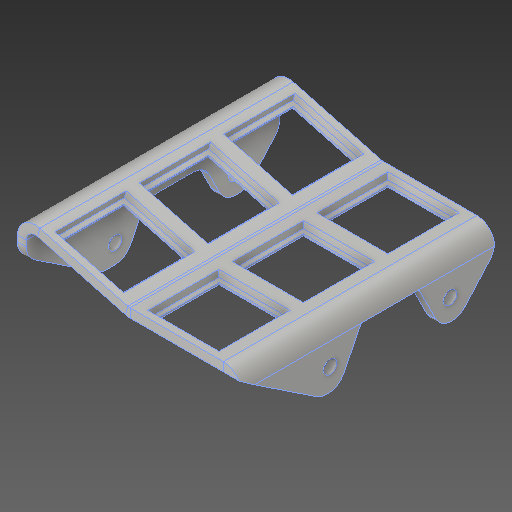
# Autodesk Inventor part: keyplate2
Saved by Autodesk Inventor 2018 (Build 220112000, 112)
## iProperties
Created: 2018-05-25
Part Number: keyplate2
Material: アルミニウム 6061
Document SubType Name: Sheet Metal
Designer: NaMACHAN
Mass: 12.3776 g
Surface Area: 65.0892 cm^2
Volume: 4.58428 cm^3
Density: 2.7 g/cm^3
Flat Pattern Width: 5.7 cm
Flat Pattern Length: 7.68162 cm
Flat Pattern Area: 43.7853 cm^2
Sheet Metal Rule: Al2mm
Sheet Metal Width: 57.000 mm
Sheet Metal Length: 76.816 mm
Sheet Metal Area: 4378.526 mm^2
Appearance: アルミニウム - フラット
Author: NaMACHAN
Autodesk Inventor part; units mm, degrees
ref_plane "YZ Plane" through (0, 0, 0) normal (1, 0, 0) x (0, 1, 0)
ref_plane "XZ Plane" through (0, 0, 0) normal (0, 1, 0) x (-1, 0, 0)
ref_plane "XY Plane" through (0, 0, 0) normal (0, 0, 1) x (1, 0, 0)
sketch "スケッチ1" plane through (0, 0, 0) normal (0, 1, 0) x (-1, 0, 0)
  line L0 (-10.5, -28.5) -> (10.5, -28.5)
  line L1 (10.5, -28.5) -> (10.5, 28.5)
  line L2 (10.5, 28.5) -> (-10.5, 28.5)
  line L3 (-10.5, 28.5) -> (-10.5, -28.5)
  line L4 (-10.5, -28.5) -> (10.5, 28.5) construction
  line L5 (10.5, -28.5) -> (-10.5, 28.5) construction
  line L6 (-7, -7) -> (7, -7)
  line L7 (7, -7) -> (7, 7)
  line L8 (7, 7) -> (-7, 7)
  line L9 (-7, 7) -> (-7, -7)
  line L10 (-7, -7) -> (7, 7) construction
  line L11 (7, -7) -> (-7, 7) construction
  line L12 (-7, -26) -> (7, -26)
  line L13 (7, -26) -> (7, -12)
  line L14 (7, -12) -> (-7, -12)
  line L15 (-7, -12) -> (-7, -26)
  line L16 (-7, -26) -> (7, -12) construction
  line L17 (7, -26) -> (-7, -12) construction
  line L18 (-7, 12) -> (7, 12)
  line L19 (7, 12) -> (7, 26)
  line L20 (7, 26) -> (-7, 26)
  line L21 (-7, 26) -> (-7, 12)
  line L22 (-7, 12) -> (7, 26) construction
  line L23 (7, 12) -> (-7, 26) construction
  point P0 (0, 0)
  point P1 (0, 0)
  point P2 (0, 0)
  point P3 (0, -19)
  point P4 (0, -19)
  point P5 (0, 19)
  point P6 (0, 19)
  point P7 (0, 0)
  dimension "d0" = 21
  dimension "d1" = 57
  dimension "d2" = 14
  dimension "d3" = 14
  dimension "d345" = 14
  dimension "d346" = 14
  dimension "d347" = 14
  dimension "d348" = 14
  dimension "d350" = 19
  dimension "d351" = 19
  measures "d0" distance of L2.end L1.end
  measures "d1" distance of L1.end L0.end
  measures "d2" distance of L8.end L7.end
  measures "d3" distance of L7.end L6.end
  measures "d345" distance of L14.end L13.end
  measures "d346" distance of L13.end L12.end
  measures "d347" distance of L20.end L19.end
  measures "d348" distance of L19.end L18.end
  measures "d350" distance of point (0, -19) point (0, 0)
  measures "d351" distance of point (0, 0) point (0, 19)
extrude "プレート1" add sketch "スケッチ1" along normal blind 2
sketch "スケッチ2" plane through (-11.0176, 2.0681, 28.5) normal (-0.258819, -0.9659258, 0) x (0.9659258, -0.258819, 0)
  line L0 (0, -57) -> (0, 0)
  line L1 (0, 0) -> (-20.4734, 0)
  line L2 (-20.4734, 0) -> (-20.4734, -57)
  line L3 (-20.4734, -57) -> (0, -57)
  constraints: 6 end point, 1 horizontal, 1 perpendicular, 1 vertical
edge flange "フランジ1" height 21 angle 15 thickness 2 bend radius 2 thickness toward (-0.258819, -0.9659258, 0) relief straight relief width 2 relief depth 1 edges at (-10.5, 2, 0) wall of the first edge with corners at (-11.0176, 2.0681, -28.5) (-11.0176, 2.0681, 28.5) (-30.7934, 7.3671, 28.5) (-30.7934, 7.3671, -28.5)
bend "曲げ1"
corner "コーナー1"
sketch "スケッチ9" plane through (-11.0176, 2.0681, 28.5) normal (0.258819, 0.9659258, 0) x (0.9659258, -0.258819, 0)
  line L0 (-17.5, 35.5) -> (-3.5, 35.5)
  line L1 (-3.5, 35.5) -> (-3.5, 21.5)
  line L2 (-3.5, 21.5) -> (-17.5, 21.5)
  line L3 (-17.5, 21.5) -> (-17.5, 35.5)
  line L4 (-17.5, 35.5) -> (-3.5, 21.5) construction
  line L5 (-3.5, 35.5) -> (-17.5, 21.5) construction
  line L6 (-20.4734, 0) -> (0, 0) projected
  line L7 (-20.4734, 57) -> (-20.4734, 0) projected
  line L8 (0, 0) -> (0, 57) projected
  line L9 (-3.5, 2.5) -> (-17.5, 2.5)
  line L10 (-17.5, 2.5) -> (-17.5, 16.5)
  line L11 (-17.5, 16.5) -> (-3.5, 16.5)
  line L12 (-3.5, 16.5) -> (-3.5, 2.5)
  line L13 (-3.5, 2.5) -> (-17.5, 16.5) construction
  line L14 (-17.5, 2.5) -> (-3.5, 16.5) construction
  line L15 (-3.5, 40.5) -> (-17.5, 40.5)
  line L16 (-17.5, 40.5) -> (-17.5, 54.5)
  line L17 (-17.5, 54.5) -> (-3.5, 54.5)
  line L18 (-3.5, 54.5) -> (-3.5, 40.5)
  line L19 (-3.5, 40.5) -> (-17.5, 54.5) construction
  line L20 (-17.5, 40.5) -> (-3.5, 54.5) construction
  point P0 (11.1775, 28.5)
  point P1 (-10.5, 28.5)
  point P2 (-10.5, 28.5)
  point P3 (-24.9734, 28.5)
  point P4 (-10.5, 28.5)
  point P5 (-10.2367, 0)
  point P6 (-17.5, 28.5)
  point P7 (-20.4734, 28.5)
  point P8 (-10.5, 9.5)
  point P9 (-10.5, 47.5)
  point P10 (-10.5, 47.5)
  point P11 (-10.5, 9.5)
  point P12 (-3.5, 9.5)
  dimension "d63" = 14
  dimension "d64" = 14
  dimension "d204" = 10.5
  dimension "d352" = 14
  dimension "d353" = 14
  dimension "d354" = 19
  dimension "d355" = 19
  constraints: 36 end point, 13 midpoint, 6 parallel, 3 horizontal, 3 perpendicular, 3 vertical alignment, 2 horizontal alignment, 1 point on line, 2 other
  measures "d63" distance of L1.end L2.end
  measures "d64" distance of L0.end L1.end
  measures "d204" distance from line of L8 point (-10.5, 28.5)
  measures "d352" distance of L15.end L16.end
  measures "d353" distance of L9.end L10.end
  measures "d354" distance of point (-10.5, 28.5) point (-10.5, 47.5)
  measures "d355" distance of point (-10.5, 9.5) point (-10.5, 28.5)
extrude "押し出し3" cut sketch "スケッチ9" against normal blind 10
sketch "スケッチ26" plane through (-33.8287, 3.5033, -28.5) normal (-1, 0, 0) x (0, -1, 0)
  line L0 (0, 57) -> (0, 0)
  line L1 (0, 0) -> (14.7871, 0)
  line L2 (14.7871, 0) -> (14.7871, 57)
  line L3 (14.7871, 57) -> (0, 57)
  constraints: 6 end point, 1 horizontal, 1 perpendicular, 1 vertical
edge flange "フランジ13" height 20 angle 105 thickness 2 bend radius 2 thickness toward (-1, 0, 0) relief straight relief width 2 relief depth 1 edges at (-31.3111, 5.4352, 0) wall of the first edge with corners at (-33.8287, 3.5033, 28.5) (-33.8287, 3.5033, -28.5) (-33.8287, -11.2838, -28.5) (-33.8287, -11.2838, 28.5)
bend "曲げ13"
corner "コーナー13"
sketch "スケッチ33" plane through (0, 2, 0) normal (0, 1, 0) x (1, 0, 0)
  line L0 (8, 8) -> (-8, 8)
  line L1 (-8, 8) -> (-8, -8)
  line L2 (-8, -8) -> (8, -8)
  line L3 (8, -8) -> (8, 8)
  line L4 (8, 8) -> (-8, -8) construction
  line L5 (-8, 8) -> (8, -8) construction
  line L6 (8, 11) -> (-8, 11)
  line L7 (-8, 11) -> (-8, 27)
  line L8 (-8, 27) -> (8, 27)
  line L9 (8, 27) -> (8, 11)
  line L10 (8, 11) -> (-8, 27) construction
  line L11 (-8, 11) -> (8, 27) construction
  line L12 (8, -27) -> (-8, -27)
  line L13 (-8, -27) -> (-8, -11)
  line L14 (-8, -11) -> (8, -11)
  line L15 (8, -11) -> (8, -27)
  line L16 (8, -27) -> (-8, -11) construction
  line L17 (-8, -27) -> (8, -11) construction
  line L18 (7, 26) -> (7, 12) projected
  line L19 (7, -12) -> (7, -26) projected
  point P0 (0, 0)
  point P1 (0, 19)
  point P2 (0, -19)
  point P3 (0, -19)
  point P4 (0, 0)
  point P5 (0, 0)
  point P6 (0, 19)
  point P7 (0, 19)
  point P8 (7, 19)
  point P9 (0, -19)
  point P10 (7, -19)
  dimension "d265" = 16
  dimension "d266" = 16
  dimension "d356" = 16
  dimension "d357" = 16
  dimension "d358" = 16
  dimension "d359" = 16
  constraints: 36 end point, 14 midpoint, 6 parallel, 3 horizontal, 3 perpendicular, 2 horizontal alignment, 2 vertical alignment
  measures "d265" distance of L2.end L1.end
  measures "d266" distance of L1.end L0.end
  measures "d356" distance of L7.end L8.end
  measures "d357" distance of L6.end L7.end
  measures "d358" distance of L13.end L14.end
  measures "d359" distance of L12.end L13.end
extrude "押し出し11" cut sketch "スケッチ33" against normal blind 1.6
sketch "スケッチ34" plane through (-11.0176, 2.0681, 28.5) normal (0.258819, 0.9659258, 0) x (0.9659258, -0.258819, 0)
  line L0 (-2.5, 36.5) -> (-18.5, 36.5)
  line L1 (-18.5, 36.5) -> (-18.5, 20.5)
  line L2 (-18.5, 20.5) -> (-2.5, 20.5)
  line L3 (-2.5, 20.5) -> (-2.5, 36.5)
  line L4 (-2.5, 36.5) -> (-18.5, 20.5) construction
  line L5 (-18.5, 36.5) -> (-2.5, 20.5) construction
  line L6 (-17.5, 21.5) -> (-17.5, 35.5) projected
  line L7 (-17.5, 35.5) -> (-3.5, 35.5) projected
  line L8 (-2.5, 1.5) -> (-18.5, 1.5)
  line L9 (-18.5, 1.5) -> (-18.5, 17.5)
  line L10 (-18.5, 17.5) -> (-2.5, 17.5)
  line L11 (-2.5, 17.5) -> (-2.5, 1.5)
  line L12 (-2.5, 1.5) -> (-18.5, 17.5) construction
  line L13 (-18.5, 1.5) -> (-2.5, 17.5) construction
  line L14 (-2.5, 39.5) -> (-18.5, 39.5)
  line L15 (-18.5, 39.5) -> (-18.5, 55.5)
  line L16 (-18.5, 55.5) -> (-2.5, 55.5)
  line L17 (-2.5, 55.5) -> (-2.5, 39.5)
  line L18 (-2.5, 39.5) -> (-18.5, 55.5) construction
  line L19 (-18.5, 39.5) -> (-2.5, 55.5) construction
  line L20 (-3.5, 16.5) -> (-3.5, 2.5) projected
  line L21 (-3.5, 54.5) -> (-3.5, 40.5) projected
  point P0 (11.1775, 28.5)
  point P1 (-10.5, 28.5)
  point P2 (-10.5, 28.5)
  point P3 (-17.5, 28.5)
  point P4 (-10.5, 28.5)
  point P5 (-10.5, 35.5)
  point P6 (-10.5, 9.5)
  point P7 (-10.5, 47.5)
  point P8 (-10.5, 47.5)
  point P9 (-10.5, 9.5)
  point P10 (-10.5, 9.5)
  point P11 (-3.5, 9.5)
  point P12 (-10.5, 47.5)
  point P13 (-3.5, 47.5)
  dimension "d269" = 16
  dimension "d270" = 16
  dimension "d360" = 16
  dimension "d361" = 16
  dimension "d362" = 16
  dimension "d363" = 16
  constraints: 36 end point, 16 midpoint, 6 parallel, 3 horizontal, 3 horizontal alignment, 3 perpendicular, 3 vertical alignment
  measures "d269" distance of L2.end L1.end
  measures "d270" distance of L1.end L0.end
  measures "d360" distance of L9.end L10.end
  measures "d361" distance of L8.end L9.end
  measures "d362" distance of L15.end L16.end
  measures "d363" distance of L14.end L15.end
extrude "押し出し12" cut sketch "スケッチ34" against normal blind 1.6
sketch "スケッチ41" plane through (12.5, -2, 28.5) normal (1, 0, 0) x (0, 1, 0)
  line L0 (0, -57) -> (0, 0)
  line L1 (0, 0) -> (-10, 0)
  line L2 (-10, 0) -> (-10, -57)
  line L3 (-10, -57) -> (0, -57)
  constraints: 6 end point, 1 horizontal, 1 perpendicular, 1 vertical
edge flange "フランジ18" height 14 angle 90 thickness 2 bend radius 2 thickness toward (1, 0, 0) relief straight relief width 2 relief depth 1 edges at (10.5, 0, 0) wall of the first edge with corners at (12.5, -2, -28.5) (12.5, -2, 28.5) (12.5, -12, 28.5) (12.5, -12, -28.5)
bend "曲げ19"
corner "コーナー18"
sketch "スケッチ43" plane through (14.5, -2, 28.5) normal (1, 0, 0) x (0, 0, -1)
  line L0 (57, -10) -> (0, -10) projected
  line L1 (57, 0) -> (57, -10) projected
  line L2 (0, -10) -> (0, 0) projected
  point P0 (28.5, 2)
  point P1 (47, -5)
  point P2 (28.5, -10)
  point P3 (49, -10)
  point P4 (8, -10)
  point P5 (57, -2)
  point P6 (20, -5)
  point P7 (0, -2)
  dimension "d337" = 5
  dimension "d364" = 10
  dimension "d365" = 20
  constraints: 1 horizontal alignment, 1 midpoint
  measures "d337" distance from line of point (47, -5) L0
  measures "d364" distance from line of L1 point (47, -5)
  measures "d365" distance from line of L2 point (20, -5)
hole "穴8" at (14.5, -7, -18.5) at (14.5, -7, 8.5) direction (-1, 0, 0) diameter 3 end through all
sketch "スケッチ45" plane through (-35.8287, -11.2838, -28.5) normal (-1, 0, 0) x (0, 0, 1)
  point P0 (28.5, 11.2838)
sketch "スケッチ46" plane through (-35.8287, -11.2838, -28.5) normal (-1, 0, 0) x (0, 0, 1)
  line L0 (0, -0.7162) -> (0, 14.7871) projected
  line L1 (12, -0.7162) -> (17, 9.2838)
  line L2 (17, 9.2838) -> (30, 9.2838)
  line L3 (30, 9.2838) -> (35, -0.7162)
  line L4 (39, -0.7162) -> (57, 11.2838)
  line L5 (57, 0) -> (57, 14.7871) projected
  line L6 (57, 11.2838) -> (57, -0.7162)
  line L7 (39, -0.7162) -> (57, -0.7162)
  line L8 (35, -0.7162) -> (12, -0.7162)
  line L9 (35.4907, -0.7162) -> (0, -0.7162)
  line L10 (0, -0.7162) -> (0, -0.7162)
  line L11 (8, -0.7162) -> (0, 8.2838)
  line L12 (0, 8.2838) -> (0, -0.7162)
  line L13 (0, -0.7162) -> (8, -0.7162)
  line L14 (0, -0.7162) -> (57, -0.7162) projected
  point P0 (28.5, 11.2838)
  dimension "d374" = 12
  dimension "d375" = 18
  dimension "d376" = 4
  dimension "d378" = 5
  dimension "d382" = 5
  dimension "d383" = 8
  dimension "d384" = 9
  dimension "d388" = 10
  dimension "d389" = 4
  constraints: 24 end point, 10 point on line, 2 collinear, 1 parallel
  measures "d374" distance of L6.end L4.end
  measures "d375" distance from line of L5 L4.start
  measures "d376" distance of L3.end L4.start
  measures "d378" horizontal distance of L1.start L1.end
  measures "d382" horizontal distance of L3.end L2.end
  measures "d383" distance of L10.end L11.start
  measures "d384" distance of L10.end L11.end
  measures "d388" distance between parallel lines of L14 L2
  measures "d389" distance of L11.start L1.start
extrude "押し出し17" cut sketch "スケッチ46" against normal blind 100
fillet "コーナーR3" radius 4 13 edges at (-34.8287, -11.2838, -21.1367) (-34.8287, -11.2838, -16.1419) (-34.8287, -2, -11.5) (-34.8287, -2, 1.5) (-34.8287, -11.2838, 6.1419) (-34.8287, -11.2838, 11.5744) (-34.8287, 0, 28.5) (13.5, -12, 10.5) (13.5, -12, 6.5) (13.5, -12, -16.5) (13.5, -12, -20.5) (13.5, -3, -28.5) (-34.8287, -3, -28.5)
equation "\"d4\" = Thickness"
equation "\"d5\" = BendReliefWidth"
equation "\"d6\" = BendReliefDepth"
equation "\"d7\" = MinimumRemnant"
equation "\"d8\" = TransitionRadius"
equation "\"d11\" = BendRadius"
equation "\"d12\" = CornerReliefSize"
equation "\"d13\" = GapSize"
equation "\"d14\" = JacobiRadiusSize"
equation "\"d205\" = BendReliefWidth"
equation "\"d206\" = BendReliefDepth"
equation "\"d207\" = MinimumRemnant"
equation "\"d208\" = TransitionRadius"
equation "\"d211\" = BendRadius"
equation "\"d212\" = CornerReliefSize"
equation "\"d213\" = GapSize"
equation "\"d214\" = JacobiRadiusSize"
equation "\"BendRadius\" = Thickness"
equation "\"BendReliefWidth\" = Thickness"
equation "\"BendReliefDepth\" = 0.5 * Thickness"
equation "\"CornerReliefSize\" = 4 * Thickness"
equation "\"MinimumRemnant\" = 2 * Thickness"
equation "\"TransitionRadius\" = BendRadius"
equation "\"JacobiRadiusSize\" = BendRadius"
equation "\"GapSize\" = Thickness"
equation "\"Thickness\" = 2"
